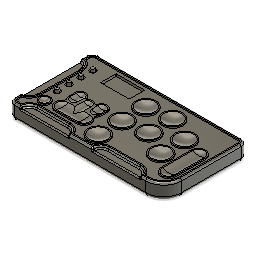
Pocket organ V11 mock-up v14 without engraving (Autodesk Fusion 360 design; units mm, degrees)
Autodesk Fusion 360 part; units mm, degrees
box "BoxPrimitive1" add length 70 width 130 height 13 placed x (0, 0, 1) y (1, 0, 0) z (0, 1, 0) at (0, 0, 0) makes body 1
fillet "Fillet1" radius 1.5 4 edges at (65, 13, 0) (130, 13, 35) (65, 13, 70) (0, 13, 35) on bodies 1
fillet "Fillet2" radius 3 4 edges at (65, 0, 70) (130, 0, 35) (65, 0, 0) (0, 0, 35) on bodies 1
fillet "Fillet3" radius 5 9 edges at (0.4393, 12.5607, 69.5607) (0, 7.25, 70) (0.8787, 0.8787, 69.1213) (0.4393, 12.5607, 0.4393) (0, 7.25, 0) (0.8787, 0.8787, 0.8787) (129.5607, 12.5607, 0.4393) (130, 7.25, 0) (129.1213, 0.8787, 0.8787) on bodies 1
fillet "Fillet4" radius 15 3 edges at (129.5607, 12.5607, 69.5607) (130, 7.25, 70) (129.1213, 0.8787, 69.1213) on bodies 1
sketch "keyboard top" plane through (0, 13, 0) normal (0, 1, 0) x (-1, 0, 0)
  arc A0 (-115, 68.5) -> (-128.5, 55) centre (-115, 55) ccw
  line L0 (-128.5, 55) -> (-128.5, 5)
  arc A1 (-128.5, 5) -> (-125, 1.5) centre (-125, 5) ccw
  line L1 (-125, 1.5) -> (-5, 1.5)
  arc A2 (-5, 1.5) -> (-1.5, 5) centre (-5, 5) ccw
  line L2 (-1.5, 5) -> (-1.5, 65)
  arc A3 (-1.5, 65) -> (-5, 68.5) centre (-5, 65) ccw
  line L3 (-5, 68.5) -> (-115, 68.5)
  line L4 (-25.5, 5) -> (-48.5, 5)
  line L5 (-49, 5.5) -> (-49, 17.5)
  line L6 (-48.5, 18) -> (-25.5, 18)
  line L7 (-25, 17.5) -> (-25, 5.5)
  line L8 (0.0001, 10) -> (0, 10)
  line L9 (-7, 17) -> (-7, 53)
  line L10 (0, 60) -> (0.0001, 60)
  arc A4 (-1.5, 59.8374) -> (-7, 53) centre (0, 53) ccw
  arc A5 (-1.5, 10.1626) -> (0, 10) centre (0, 17) ccw
  line L11 (0, 0) -> (-130, 0)
  line L12 (-130, 0) -> (-130, 70)
  line L13 (-130, 70) -> (0, 70)
  line L14 (0, 70) -> (0, 0)
  arc A6 (-49, 5.5) -> (-48.5, 5) centre (-48.5, 5.5) ccw
  arc A7 (-48.5, 18) -> (-49, 17.5) centre (-48.5, 17.5) ccw
  arc A8 (-25, 17.5) -> (-25.5, 18) centre (-25.5, 17.5) ccw
  arc A9 (-25.5, 5) -> (-25, 5.5) centre (-25.5, 5.5) ccw
  line L15 (-10, 69.9) -> (-10, 70)
  line L16 (-16.9, 63) -> (-43.1, 63)
  line L17 (-50, 69.9) -> (-50, 70)
  line L18 (-70, 69.9) -> (-70, 70)
  line L19 (-76.9, 63) -> (-103.1, 63)
  line L20 (-110, 69.9) -> (-110, 70)
  arc A10 (-110, 69.9) -> (-109.8565, 68.5) centre (-103.1, 69.9) ccw
  arc A11 (-76.9, 63) -> (-70.1435, 68.5) centre (-76.9, 69.9) ccw
  arc A12 (-50, 69.9) -> (-49.8565, 68.5) centre (-43.1, 69.9) ccw
  arc A13 (-10.1435, 68.5) -> (-10, 69.9) centre (-16.9, 69.9) ccw
  line L21 (-7, 0) -> (-13, 0)
  line L22 (-13, 0) -> (-13, 12.5)
  line L23 (-13, 12.5) -> (-13, 22.5)
  line L24 (-13, 22.5) -> (-13, 32.5)
  circle A14 centre (-13, 12.5) radius 2.5
  circle A15 centre (-13, 22.5) radius 2.5
  circle A16 centre (-13, 32.5) radius 2.5
  line L25 (-13, 32.5) -> (-13, 42.5)
  circle A17 centre (-13, 42.5) radius 2.5
  circle A18 centre (-13, 12.5) radius 1.5
  circle A19 centre (-13, 22.5) radius 1.5
  circle A20 centre (-13, 32.5) radius 1.5
  circle A21 centre (-13, 42.5) radius 1.5
  line L26 (-130, 0) -> (-102.5, 0)
  line L27 (-102.5, 0) -> (-82.5, 0)
  line L28 (-82.5, 0) -> (-62.5, 0)
  line L29 (-130, 0) -> (-119, 0)
  line L30 (-102.5, 0) -> (-102.5, 25)
  line L31 (-102.5, 25) -> (-102.5, 45)
  circle A22 centre (-102.5, 25) radius 7.5
  circle A23 centre (-102.5, 45) radius 7.5
  line L32 (-82.5, 0) -> (-82.5, 15)
  line L33 (-82.5, 15) -> (-82.5, 35)
  line L34 (-62.5, 0) -> (-62.5, 17.5)
  line L35 (-62.5, 17.5) -> (-62.5, 37.5)
  line L36 (-62.5, 37.5) -> (-62.5, 57.5)
  circle A24 centre (-82.5, 15) radius 7.5
  circle A25 centre (-82.5, 35) radius 7.5
  circle A26 centre (-62.5, 17.5) radius 7.5
  circle A27 centre (-62.5, 37.5) radius 7.5
  circle A28 centre (-62.5, 57.5) radius 7.5
  line L37 (-119, 30) -> (-119, 55) construction
  line L38 (0, 0) -> (-27, 0)
  line L39 (-27, 52) -> (-45, 52)
  line L40 (-27, 57) -> (-45, 57)
  arc A29 (-45, 57) -> (-45, 47) centre (-45, 52) ccw
  line L41 (-39.5, 47) -> (-32.5, 47)
  arc A30 (-27, 47) -> (-27, 57) centre (-27, 52) ccw
  line L42 (-27, 52) -> (-45, 52) construction
  line L43 (-36, 52) -> (-36, 40)
  line L44 (-45, 37) -> (-45, 42)
  line L45 (-27, 37) -> (-27, 42)
  line L46 (-32.5, 40) -> (-32.5, 47)
  arc A31 (-32.5, 52) -> (-39.5, 52) centre (-36, 52) ccw
  line L47 (-39.5, 52) -> (-39.5, 47)
  arc A32 (-39.5, 40) -> (-32.5, 40) centre (-36, 40) ccw
  line L48 (-36, 40) -> (-36, 52) construction
  line L49 (-41.5, 37) -> (-41.5, 42)
  arc A33 (-41.5, 42) -> (-48.5, 42) centre (-45, 42) ccw
  line L50 (-48.5, 42) -> (-48.5, 37)
  arc A34 (-48.5, 37) -> (-41.5, 37) centre (-45, 37) ccw
  line L51 (-45, 37) -> (-45, 42) construction
  line L52 (-23.5, 37) -> (-23.5, 42)
  arc A35 (-23.5, 42) -> (-30.5, 42) centre (-27, 42) ccw
  line L53 (-30.5, 42) -> (-30.5, 37)
  arc A36 (-30.5, 37) -> (-23.5, 37) centre (-27, 37) ccw
  line L54 (-27, 37) -> (-27, 42) construction
  line L55 (-114, 30) -> (-114, 55)
  arc A37 (-114, 55) -> (-124, 55) centre (-119, 55) ccw
  line L56 (-124, 55) -> (-124, 30)
  arc A38 (-124, 30) -> (-114, 30) centre (-119, 30) ccw
  line L57 (-119, 30) -> (-119, 55) construction
  line L58 (-27, 52) -> (-15, 52)
  line L59 (-15, 52) -> (-15, 55)
  circle A39 centre (-15, 55) radius 3.5
  line L60 (-119, 55) -> (-119, 30)
  line L61 (-45, 37) -> (-45, 42)
  line L62 (-27, 37) -> (-27, 42)
  line L63 (-49.8565, 68.5) -> (-70.1435, 68.5)
  line L64 (-109.8565, 68.5) -> (-115, 68.5)
  line L65 (-128.5, 55) -> (-128.5, 5)
  line L66 (-125, 1.5) -> (-5, 1.5)
  line L67 (-1.5, 10.1626) -> (-1.5, 5)
  line L68 (-1.5, 59.8374) -> (-1.5, 65)
  line L69 (-10.1435, 68.5) -> (-5, 68.5)
  arc A40 (-1.5, 65) -> (-5, 68.5) centre (-5, 65) ccw
  arc A41 (-5, 1.5) -> (-1.5, 5) centre (-5, 5) ccw
  arc A42 (-128.5, 5) -> (-125, 1.5) centre (-125, 5) ccw
  arc A43 (-115, 68.5) -> (-128.5, 55) centre (-115, 55) ccw
  arc A44 (-109.8565, 68.5) -> (-103.1, 63) centre (-103.1, 69.9) ccw
  arc A45 (-70.1435, 68.5) -> (-70, 69.9) centre (-76.9, 69.9) ccw
  arc A46 (-49.8565, 68.5) -> (-43.1, 63) centre (-43.1, 69.9) ccw
  arc A47 (-16.9, 63) -> (-10.1435, 68.5) centre (-16.9, 69.9) ccw
  arc A48 (0, 60) -> (-1.5, 59.8374) centre (0, 53) ccw
  arc A49 (-7, 17) -> (-1.5, 10.1626) centre (0, 17) ccw
  arc A50 (-110.6266, 67.5) -> (-103.1, 62) centre (-103.1, 69.9) ccw
  line L70 (-76.9, 62) -> (-103.1, 62)
  arc A51 (-76.9, 62) -> (-69.3734, 67.5) centre (-76.9, 69.9) ccw
  line L71 (-50.6266, 67.5) -> (-69.3734, 67.5)
  arc A52 (-50.6266, 67.5) -> (-43.1, 62) centre (-43.1, 69.9) ccw
  line L72 (-16.9, 62) -> (-43.1, 62)
  arc A53 (-16.9, 62) -> (-9.3734, 67.5) centre (-16.9, 69.9) ccw
  line L73 (-9.3734, 67.5) -> (-5, 67.5)
  arc A54 (-2.5, 65) -> (-5, 67.5) centre (-5, 65) ccw
  line L74 (-2.5, 60.5993) -> (-2.5, 65)
  arc A55 (-2.5, 60.5993) -> (-8, 53) centre (0, 53) ccw
  line L75 (-8, 17) -> (-8, 53)
  arc A56 (-8, 17) -> (-2.5, 9.4007) centre (0, 17) ccw
  line L76 (-2.5, 9.4007) -> (-2.5, 5)
  arc A57 (-5, 2.5) -> (-2.5, 5) centre (-5, 5) ccw
  line L77 (-125, 2.5) -> (-5, 2.5)
  arc A58 (-127.5, 5) -> (-125, 2.5) centre (-125, 5) ccw
  line L78 (-127.5, 55) -> (-127.5, 5)
  arc A59 (-115, 67.5) -> (-127.5, 55) centre (-115, 55) ccw
  line L79 (-110.6266, 67.5) -> (-115, 67.5)
  line L80 (-125, 55) -> (-125, 30)
  arc A60 (-125, 30) -> (-113, 30) centre (-119, 30) ccw
  line L81 (-113, 30) -> (-113, 55)
  arc A61 (-113, 55) -> (-125, 55) centre (-119, 55) ccw
  circle A62 centre (-102.5, 25) radius 8.5
  circle A63 centre (-102.5, 45) radius 8.5
  circle A64 centre (-82.5, 35) radius 8.5
  circle A65 centre (-82.5, 15) radius 8.5
  circle A66 centre (-62.5, 17.5) radius 8.5
  circle A67 centre (-62.5, 37.5) radius 8.5
  circle A68 centre (-62.5, 57.5) radius 8.5
  line L82 (-40.5, 40) -> (-40.5, 42)
  arc A69 (-40.5, 42) -> (-46.5827, 46.2125) centre (-45, 42) ccw
  line L83 (-49.5, 42) -> (-49.5, 37)
  arc A70 (-49.5, 37) -> (-40.5, 37) centre (-45, 37) ccw
  arc A71 (-25.4173, 46.2125) -> (-31.5, 42) centre (-27, 42) ccw
  line L84 (-31.5, 42) -> (-31.5, 40)
  arc A72 (-31.5, 37) -> (-22.5, 37) centre (-27, 37) ccw
  line L85 (-22.5, 37) -> (-22.5, 42)
  circle A73 centre (-15, 55) radius 4.5
  line L86 (-39.5, 47) -> (-39.5, 40)
  line L87 (-32.5, 47) -> (-32.5, 52)
  line L88 (-32.5, 47) -> (-27, 47)
  line L89 (-45, 47) -> (-39.5, 47)
  line L90 (-40.5, 46) -> (-40.5, 40)
  line L91 (-31.5, 40) -> (-31.5, 46)
  line L92 (-31.5, 46) -> (-27, 46)
  line L93 (-27, 58) -> (-45, 58)
  arc A74 (-46.5827, 46.2125) -> (-45, 46) centre (-45, 52) ccw
  line L94 (-45, 46) -> (-40.5, 46)
  arc A75 (-45, 58) -> (-48.893, 47.4344) centre (-45, 52) ccw
  arc A76 (-48.5935, 44.7087) -> (-49.5, 42) centre (-45, 42) ccw
  line L95 (-40.5, 37) -> (-40.5, 40)
  line L96 (-31.5, 40) -> (-31.5, 37)
  arc A77 (-27, 46) -> (-25.4173, 46.2125) centre (-27, 52) ccw
  arc A78 (-21, 52) -> (-27, 58) centre (-27, 52) ccw
  arc A79 (-23.107, 47.4344) -> (-21, 52) centre (-27, 52) ccw
  arc A80 (-22.5, 42) -> (-23.4065, 44.7087) centre (-27, 42) ccw
  arc A81 (-23.107, 47.4344) -> (-23.4065, 44.7087) centre (-21.8094, 45.9125) ccw
  arc A82 (-48.5935, 44.7087) -> (-48.893, 47.4344) centre (-50.1906, 45.9125) ccw
  line L97 (-31.5, 37) -> (-32.6459, 37)
  line L98 (-40.5, 37) -> (-39.3541, 37)
  arc A83 (-40.5, 40) -> (-39.3541, 37) centre (-36, 40) ccw
  arc A84 (-32.6459, 37) -> (-31.5, 40) centre (-36, 40) ccw
  arc A85 (-39.3541, 37) -> (-32.6459, 37) centre (-36, 40) ccw
  arc A86 (-111.6703, 67.5) -> (-103.1, 61) centre (-103.1, 69.9) ccw
  line L99 (-76.9, 61) -> (-103.1, 61)
  arc A87 (-76.9, 61) -> (-68.3297, 67.5) centre (-76.9, 69.9) ccw
  arc A88 (-51.6703, 67.5) -> (-43.1, 61) centre (-43.1, 69.9) ccw
  line L100 (-16.9, 61) -> (-43.1, 61)
  arc A89 (-16.9, 61) -> (-8.3297, 67.5) centre (-16.9, 69.9) ccw
  arc A90 (-2.5, 61.6458) -> (-9, 53) centre (0, 53) ccw
  line L101 (-9, 17) -> (-9, 53)
  arc A91 (-9, 17) -> (-2.5, 8.3542) centre (0, 17) ccw
  line L102 (-28.4325, 53.5487) -> (-44.8065, 53.5487) construction
  line L103 (-44.8065, 53.5487) -> (-44.8065, 47.5487) construction
  line L104 (-44.8065, 47.5487) -> (-28.4325, 47.5487) construction
  line L105 (-28.4325, 47.5487) -> (-28.4325, 53.5487) construction
  line L106 (-59.4724, 21.1298) -> (-65.7077, 21.1298) construction
  line L107 (-65.7077, 21.1298) -> (-65.7077, 11.1298) construction
  line L108 (-65.7077, 11.1298) -> (-59.4724, 11.1298) construction
  line L109 (-59.4724, 11.1298) -> (-59.4724, 21.1298) construction
  line L110 (-79.7168, 18.5949) -> (-85.7178, 18.5949) construction
  line L111 (-85.7178, 18.5949) -> (-85.7178, 8.5949) construction
  line L112 (-85.7178, 8.5949) -> (-79.7168, 8.5949) construction
  line L113 (-79.7168, 8.5949) -> (-79.7168, 18.5949) construction
  line L114 (-99.8243, 28.6873) -> (-105.2686, 28.6873) construction
  line L115 (-105.2686, 28.6873) -> (-105.2686, 18.6873) construction
  line L116 (-105.2686, 18.6873) -> (-99.8243, 18.6873) construction
  line L117 (-99.8243, 18.6873) -> (-99.8243, 28.6873) construction
  line L118 (-60.2821, 41.2383) -> (-65.1893, 41.2383) construction
  line L119 (-65.1893, 41.2383) -> (-65.1893, 31.2383) construction
  line L120 (-65.1893, 31.2383) -> (-60.2821, 31.2383) construction
  line L121 (-60.2821, 31.2383) -> (-60.2821, 41.2383) construction
  line L122 (-79.041, 38.5391) -> (-85.7354, 38.5391) construction
  line L123 (-85.7354, 38.5391) -> (-85.7354, 28.5391) construction
  line L124 (-85.7354, 28.5391) -> (-79.041, 28.5391) construction
  line L125 (-79.041, 28.5391) -> (-79.041, 38.5391) construction
  line L126 (-98.874, 48.4203) -> (-106.0566, 48.4203) construction
  line L127 (-106.0566, 48.4203) -> (-106.0566, 38.4203) construction
  line L128 (-106.0566, 38.4203) -> (-98.874, 38.4203) construction
  line L129 (-98.874, 38.4203) -> (-98.874, 48.4203) construction
  line L130 (-59.6073, 61.3467) -> (-65.6034, 61.3467) construction
  line L131 (-65.6034, 61.3467) -> (-65.6034, 51.3467) construction
  line L132 (-65.6034, 51.3467) -> (-59.6073, 51.3467) construction
  line L133 (-59.6073, 51.3467) -> (-59.6073, 61.3467) construction
  line L134 (-116.6195, 46.4025) -> (-121.9759, 46.4025) construction
  line L135 (-121.9759, 46.4025) -> (-121.9759, 36.4025) construction
  line L136 (-121.9759, 36.4025) -> (-116.6195, 36.4025) construction
  line L137 (-116.6195, 36.4025) -> (-116.6195, 46.4025) construction
  line L138 (-14.0627, 56.7468) -> (-16.382, 56.7468) construction
  line L139 (-16.382, 56.7468) -> (-16.382, 51.7468) construction
  line L140 (-16.382, 51.7468) -> (-14.0627, 51.7468) construction
  line L141 (-14.0627, 51.7468) -> (-14.0627, 56.7468) construction
  line L142 (-25.6408, 36.5912) -> (-25.6408, 42.4115) construction
  line L143 (-25.6408, 42.4115) -> (-29.6408, 42.4115) construction
  line L144 (-29.6408, 42.4115) -> (-29.6408, 36.5912) construction
  line L145 (-29.6408, 36.5912) -> (-25.6408, 36.5912) construction
  line L146 (-34.3337, 38.9989) -> (-34.3337, 44.5516) construction
  line L147 (-34.3337, 44.5516) -> (-38.3337, 44.5516) construction
  line L148 (-38.3337, 44.5516) -> (-38.3337, 38.9989) construction
  line L149 (-38.3337, 38.9989) -> (-34.3337, 38.9989) construction
  line L150 (-43.8694, 36.5932) -> (-43.8694, 42.1537) construction
  line L151 (-43.8694, 42.1537) -> (-47.8694, 42.1537) construction
  line L152 (-47.8694, 42.1537) -> (-47.8694, 36.5932) construction
  line L153 (-47.8694, 36.5932) -> (-43.8694, 36.5932) construction
  point P0 (-25, 5)
  point P1 (-49, 5)
  point P2 (-25, 18)
  point P3 (-10, 63)
  point P4 (-50, 63)
  point P5 (-70, 63)
  point P6 (-110, 63)
  dimension "d10" = 24
  dimension "d11" = 13
  dimension "d12" = 7
  dimension "d13" = 7
  dimension "d18" = 0.5
  dimension "d21" = 40
  dimension "d22" = 40
  dimension "d23" = 6.9
  dimension "d28" = 6
  dimension "d29" = 12.5
  dimension "d30" = 10
  dimension "d31" = 10
  dimension "d32" = 5
  dimension "d33" = 5
  dimension "d34" = 5
  dimension "d35" = 10
  dimension "d36" = 5
  dimension "d37" = 3
  dimension "d38" = 3
  dimension "d39" = 3
  dimension "d40" = 3
  dimension "d46" = 27.5
  dimension "d47" = 20
  dimension "d48" = 20
  dimension "d49" = 11
  dimension "d50" = 55
  dimension "d51" = 25
  dimension "d52" = 20
  dimension "d53" = 15
  dimension "d54" = 15
  dimension "d55" = 15
  dimension "d56" = 20
  dimension "d57" = 17.5
  dimension "d58" = 20
  dimension "d59" = 20
  dimension "d60" = 15
  dimension "d61" = 15
  dimension "d62" = 15
  dimension "d63" = 15
  dimension "d64" = 15
  dimension "d65" = 30
  dimension "d74" = 27
  dimension "d75" = 52
  dimension "d76" = 18
  dimension "d77" = 10
  dimension "d78" = 15
  dimension "d79" = 5
  dimension "d80" = 15
  dimension "d81" = 5
  dimension "d82" = 7
  dimension "d83" = 7
  dimension "d84" = 7
  dimension "d86" = 10
  dimension "d87" = 7
  dimension "d120" = 1
  dimension "d121" = 1
  dimension "d122" = 1
  dimension "d123" = 1
  dimension "d124" = 1
  dimension "d125" = 1
  dimension "d126" = 1
  dimension "d127" = 1
  dimension "d128" = 1
  dimension "d131" = 1
  dimension "d133" = 2
  dimension "d134" = 2
  constraint horizontal L4
  constraint vertical L5
  constraint horizontal L6
  constraint vertical L7
  constraint tangent L9 A4
  constraint tangent L10 A4
  constraint tangent L8 A5
  constraint tangent L9 A5
  constraint horizontal L11
  constraint vertical L12
  constraint horizontal L13
  constraint vertical L14
  constraint coincident L11.start L14.end
  constraint coincident P1 L4
  constraint coincident P1 L5
  constraint tangent L4 A6
  constraint tangent L5 A6
  constraint tangent L5 A7
  constraint tangent L6 A7
  constraint equal A6 A7
  constraint coincident P2 L6
  constraint coincident P2 L7
  constraint tangent L6 A8
  constraint tangent L7 A8
  constraint equal A6 A8
  constraint coincident P0 L4
  constraint coincident P0 L7
  constraint tangent L4 A9
  constraint tangent L7 A9
  constraint equal A6 A9
  constraint coincident L13 L15.end
  constraint perpendicular L13 L15
  constraint perpendicular L15 L16
  constraint coincident L13 L17.end
  constraint perpendicular L13 L17
  constraint coincident L13 L18.end
  constraint perpendicular L13 L18
  constraint horizontal L19
  constraint coincident L13 L20.end
  constraint perpendicular L13 L20
  constraint coincident P6 L19
  constraint coincident P6 L20
  constraint tangent L19 A10
  constraint tangent L20 A10
  constraint coincident P5 L18
  constraint coincident P5 L19
  constraint tangent L18 A11
  constraint tangent L19 A11
  constraint equal A10 A11
  constraint coincident P4 L16
  constraint coincident P4 L17
  constraint tangent L16 A12
  constraint tangent L17 A12
  constraint equal A10 A12
  constraint coincident P3 L15
  constraint coincident P3 L16
  constraint tangent L15 A13
  constraint tangent L16 A13
  constraint equal A10 A13
  constraint coincident L11 L21.start
  constraint coincident L11 L21.end
  constraint perpendicular L21 L22
  constraint perpendicular L1 L23
  constraint coincident L22.end L23.start
  constraint coincident L23.end L24.start
  constraint coincident L24.end A16.centre
  constraint coincident L25.end A17.centre
  constraint concentric A14 A18
  constraint concentric A15 A19
  constraint concentric A16 A20
  constraint concentric A17 A21
  constraint perpendicular L12 L26
  constraint parallel L11 L27
  constraint parallel L11 L28
  constraint perpendicular L12 L29
  constraint perpendicular L1 L30
  constraint coincident L30.end L31.start
  constraint coincident L31.end A23.centre
  constraint perpendicular L1 L32
  constraint perpendicular L11 L34
  constraint coincident L32.end L33.start
  constraint coincident L33.end A25.centre
  constraint coincident L34.end L35.start
  constraint coincident L35.end L36.start
  constraint coincident L36.end A28.centre
  constraint perpendicular L14 L38
  constraint tangent L40 A29
  constraint tangent A29 L41
  constraint parallel L40 L41
  constraint tangent L41 A30
  constraint tangent L40 A30
  constraint coincident L39.end A29.centre
  constraint coincident L39.start A30.centre
  constraint midpoint L39 L43.start
  constraint perpendicular L39 L43
  constraint tangent L46 A31
  constraint tangent A31 L47
  constraint parallel L46 L47
  constraint tangent L47 A32
  constraint tangent L46 A32
  constraint coincident L43.start A31.centre
  constraint perpendicular L39 L48
  constraint coincident L43.end A32.centre
  constraint tangent L49 A33
  constraint tangent A33 L50
  constraint parallel L49 L50
  constraint tangent L50 A34
  constraint tangent L49 A34
  constraint coincident L44.end A33.centre
  constraint coincident L44.start A34.centre
  constraint tangent L52 A35
  constraint tangent A35 L53
  constraint parallel L52 L53
  constraint tangent L53 A36
  constraint tangent L52 A36
  constraint coincident L45.end A35.centre
  constraint coincident L45.start A36.centre
  constraint tangent L55 A37
  constraint tangent A37 L56
  constraint parallel L55 L56
  constraint tangent L56 A38
  constraint tangent L55 A38
  constraint coincident L37.end A37.centre
  constraint coincident L37.start A38.centre
  constraint perpendicular L58 L59
  constraint coincident L59.end A39.centre
  constraint coincident L3 A12.end
  constraint coincident L3 A11.end
  constraint coincident L3 A10.end
  constraint coincident A0.start L3.end
  constraint coincident A0.end L0.start
  constraint coincident L0.end A1.start
  constraint coincident A1.end L1.start
  constraint coincident L1.end A2.start
  constraint coincident L2 A5.start
  constraint coincident A2.end L2.start
  constraint coincident L2 A4.start
  constraint coincident L2.end A3.start
  constraint coincident L3 A13.start
  constraint coincident A3.end L3.start
  constraint tangent L0 A42
  constraint tangent L64 A43
  constraint concentric A10 A44
  constraint concentric A11 A45
  constraint concentric A12 A46
  constraint concentric A13 A47
  constraint concentric A4 A48
  constraint concentric A5 A49
  constraint tangent A31 L86
  constraint parallel L46 L86
  constraint parallel L47 L87
  constraint tangent A29 L88
  constraint parallel L40 L89
  constraint parallel L86 L90
  constraint concentric A32 A83
  constraint parallel L46 L91
  constraint parallel L88 L92
  constraint concentric A30 A77
  constraint parallel L40 L93
  constraint concentric A29 A74
  constraint parallel L89 L94
  constraint tangent L91 A83
  constraint tangent L90 A83
  constraint tangent A74 L94
  constraint tangent L92 A77
  constraint tangent L93 A77
  constraint tangent L93 A74
  constraint concentric A74 A75
  constraint parallel L49 L82
  constraint concentric A33 A69
  constraint parallel L50 L83
  constraint concentric A34 A70
  constraint tangent L82 A70
  constraint tangent L82 A69
  constraint tangent A69 L83
  constraint tangent L83 A70
  constraint concentric A69 A76
  constraint parallel L49 L95
  constraint tangent A69 L95
  constraint concentric A35 A71
  constraint parallel L53 L84
  constraint concentric A36 A72
  constraint parallel L52 L85
  constraint tangent A71 L85
  constraint tangent L84 A72
  constraint tangent A71 L84
  constraint tangent A72 L85
  constraint parallel L53 L96
  constraint tangent A71 L96
  constraint coincident L58 A78.start
  constraint concentric A77 A78
  constraint concentric A77 A79
  constraint concentric A71 A80
  constraint tangent A80 A81
  constraint tangent A79 A81
  constraint tangent A76 A82
  constraint tangent A75 A82
  constraint coincident L97.end A83
  constraint perpendicular L96 L97
  constraint perpendicular L95 L98
  constraint concentric A83 A84
  constraint concentric A83 A85
  constraint concentric A4 A90
  constraint parallel L9 L101
  constraint concentric A49 A91
  constraint tangent L101 A91
  constraint tangent A90 L101
  constraint coincident L76 A91.end
  constraint coincident L74 A90.start
  constraint concentric A46 A88
  constraint parallel L16 L100
  constraint concentric A47 A89
  constraint tangent A88 L100
  constraint tangent L100 A89
  constraint coincident L73 A89.end
  constraint coincident L71 A88.start
  constraint concentric A44 A86
  constraint parallel L19 L99
  constraint concentric A11 A87
  constraint tangent A86 L99
  constraint tangent L99 A87
  constraint coincident L71 A87.end
  constraint coincident L79 A86.start
  constraint perpendicular L102 L103
  constraint parallel L102 L104
  constraint parallel L103 L105
  constraint perpendicular L106 L107
  constraint parallel L106 L108
  constraint parallel L107 L109
  constraint perpendicular L110 L111
  constraint parallel L110 L112
  constraint parallel L111 L113
  constraint perpendicular L114 L115
  constraint parallel L114 L116
  constraint parallel L115 L117
  constraint perpendicular L118 L119
  constraint parallel L118 L120
  constraint parallel L119 L121
  constraint perpendicular L122 L123
  constraint parallel L122 L124
  constraint parallel L123 L125
  constraint perpendicular L126 L127
  constraint parallel L126 L128
  constraint parallel L127 L129
  constraint perpendicular L130 L131
  constraint parallel L130 L132
  constraint parallel L131 L133
  constraint perpendicular L134 L135
  constraint parallel L134 L136
  constraint parallel L135 L137
  constraint perpendicular L138 L139
  constraint parallel L138 L140
  constraint parallel L139 L141
  constraint perpendicular L142 L143
  constraint parallel L142 L144
  constraint parallel L143 L145
  constraint perpendicular L146 L147
  constraint parallel L146 L148
  constraint parallel L147 L149
  constraint perpendicular L150 L151
  constraint parallel L150 L152
  constraint parallel L151 L153
  measures "d10" distance of P0 P1
  measures "d11" distance of P0 P2
  measures "d12" radius of A4
  measures "d13" radius of A5
  measures "d18" radius of A6
  measures "d21" distance of P3 P4
  measures "d22" distance of P5 P6
  measures "d23" radius of A10
  measures "d28" distance of L21.start L21.end
  measures "d29" distance of L21.end L22.end
  measures "d30" distance of L22.end L23.end
  measures "d31" distance of L23.end L24.end
  measures "d32" diameter of A14
  measures "d33" diameter of A15
  measures "d34" diameter of A16
  measures "d35" distance of L24.end L25.end
  measures "d36" diameter of A17
  measures "d37" diameter of A18
  measures "d38" diameter of A19
  measures "d39" diameter of A20
  measures "d40" diameter of A21
  measures "d46" distance of L11.end L26.end
  measures "d47" distance of L26.end L27.end
  measures "d48" distance of L27.end L28.end
  measures "d49" distance of L11.end L29.end
  measures "d50" distance of L29.end L37.end
  measures "d51" distance of L26.end L30.end
  measures "d52" distance of L30.end L31.end
  measures "d53" diameter of A22
  measures "d54" diameter of A23
  measures "d55" distance of L27.end L32.end
  measures "d56" distance of L32.end L33.end
  measures "d57" distance of L28.end L34.end
  measures "d58" distance of L34.end L35.end
  measures "d59" distance of L35.end L36.end
  measures "d60" diameter of A24
  measures "d61" diameter of A25
  measures "d62" diameter of A26
  measures "d63" diameter of A27
  measures "d64" diameter of A28
  measures "d65" distance of L29.end L37.start
  measures "d74" distance of L11.start L38.end
  measures "d75" distance of L38.end L39.start
  measures "d76" distance of L39.start L39.end
  measures "d77" diameter of A29
  measures "d78" distance of L39.end L44.start
  measures "d79" distance of L44.start L44.end
  measures "d80" distance of L39.start L45.start
  measures "d81" distance of L45.start L45.end
  measures "d82" diameter of A31
  measures "d83" diameter of A33
  measures "d84" diameter of A35
  measures "d86" diameter of A37
  measures "d87" diameter of A39
  measures "d133" radius of A81
  measures "d134" radius of A82
extrude "Extrude1" cut sketch "keyboard top" against normal blind 2 contours L2 A5 L14 A48 | L2 L9 A4 A49 bodies 1
fillet "Fillet5" radius 1 8 edges at (0, 11.25, 10) (0.4432, 12.5645, 10.014) (5.4544, 13, 12.6125) (7, 13, 35) (5.4544, 13, 57.3875) (0.4432, 12.5645, 59.986) (0, 11.25, 60) (0, 11, 35) on bodies 1
fillet "Fillet6" radius 1 7 edges at (0.25, 10.6614, 9.7242) (0.938, 10.998, 10.0631) (5.2915, 11, 12.4174) (7, 11, 35) (5.2915, 11, 57.5826) (0.938, 10.998, 59.9369) (0.25, 10.6614, 60.2758) on bodies 1
extrude "Extrude2" cut sketch "keyboard top" against normal blind 3 contours L4 L5 L6 L7 A6 A7 A8 A9 bodies 1
extrude "Extrude3" cut sketch "keyboard top" against normal blind 2 contours L3 L13 L18 L20 A10 A45 | L3 L19 A11 A44 | L3 L13 L15 L17 A12 A13 | L3 L16 A46 A47 bodies 1
fillet "Fillet7" radius 1 20 edges at (10, 11.25, 70) (10, 11.7739, 69.9748) (10.0221, 12.7363, 69.3487) (12.544, 13, 64.5488) (30, 13, 63) (47.456, 13, 64.5488) (49.9779, 12.7363, 69.3487) (50, 11.7739, 69.9748) (50, 11.25, 70) (30, 11, 70) (70, 11.25, 70) (70, 11.7739, 69.9748) (70.0221, 12.7363, 69.3487) (72.544, 13, 64.5488) (90, 13, 63) (107.456, 13, 64.5488) (109.9779, 12.7363, 69.3487) (110, 11.7739, 69.9748) (110, 11.25, 70) (90, 11, 70) on bodies 1
fillet "Fillet8" radius 1 14 edges at (9.717, 10.6656, 69.7463) (10.0518, 10.9984, 69.0566) (12.3503, 11, 64.7125) (30, 11, 63) (47.6497, 11, 64.7125) (49.9482, 10.9984, 69.0566) (50.283, 10.6656, 69.7463) (69.717, 10.6656, 69.7463) (70.0518, 10.9984, 69.0566) (72.3503, 11, 64.7125) (90, 11, 63) (107.6497, 11, 64.7125) (109.9482, 10.9984, 69.0566) (110.283, 10.6656, 69.7463) on bodies 1
extrude "Extrude4" cut sketch "keyboard top" against normal blind 1.5 contours L22 L23 A14 A18 | L22 L23 A14 A18 | L23 L24 A15 A19 | L23 L24 A15 A19 | L24 A16 L25 A20 | L24 A16 L25 A20 | A17 bodies 1
extrude "Extrude5" add sketch "keyboard top" along normal blind 2 contours L22 L23 A18 | L22 L23 A18 | L23 L24 A19 | L23 L24 A19 | L24 L25 A20 | L24 L25 A20 | A21 bodies 1
fillet "Fillet9" radius 1 4 edges at (14.3985, 15, 11.9576) (14.3985, 15, 21.9576) (14.3985, 15, 31.9576) (14.3985, 15, 41.9576) on bodies 1
sphere "SpherePrimitive1" add diameter 39 placed x (-1, 0, 0) y (0, 0, 1) z (0, 1, 0) at (62.5, 13, 17.5) separate body makes body 2
sphere "SpherePrimitive2" add diameter 39 placed x (-1, 0, 0) y (0, 0, 1) z (0, 1, 0) at (62.5, 13, 37.5) bodies 2
sphere "SpherePrimitive3" add diameter 39 placed x (-1, 0, 0) y (0, 0, 1) z (0, 1, 0) at (62.5, 13, 57.5) bodies 2
sphere "SpherePrimitive4" add diameter 39 placed x (-1, 0, 0) y (0, 0, 1) z (0, 1, 0) at (82.5, 13, 15) bodies 2
sphere "SpherePrimitive5" add diameter 39 placed x (-1, 0, 0) y (0, 0, 1) z (0, 1, 0) at (82.5, 13, 35) bodies 2
sphere "SpherePrimitive6" add diameter 39 placed x (-1, 0, 0) y (0, 0, 1) z (0, 1, 0) at (102.5, 13, 25) bodies 2
sphere "SpherePrimitive7" add diameter 39 placed x (-1, 0, 0) y (0, 0, 1) z (0, 1, 0) at (102.5, 13, 45) bodies 2
move_body "Move1" bodies 2 to x (1, 0, 0) y (0, 1, 0) z (0, 0, 1) at (0, 18, 0)
combine "Combine1" operation cut target body 1 tool bodies 2 keep tools
sphere "SpherePrimitive9" add diameter 26 placed x (-1, 0, 0) y (0, 0, 1) z (0, 1, 0) at (119, 13, 55) separate body makes body 3
sphere "SpherePrimitive10" add diameter 26 placed x (-1, 0, 0) y (0, 0, 1) z (0, 1, 0) at (119, 13, 30) separate body makes body 4
pipe "Pipe1" add diameter 26 path "keyboard top" along L60 bodies 3 4 merging no bodies
combine "Combine2" operation add target body 3 tool bodies 4 keep tools
combine "Combine3" operation add target body 3 tool bodies 4
move_body "Move2" bodies 3 to x (1, 0, 0) y (0, 1, 0) z (0, 0, 1) at (0, 12, 0)
combine "Combine4" operation cut target body 1 tool bodies 3 keep tools
sphere "SpherePrimitive11" add diameter 26 placed x (-1, 0, 0) y (0, 0, 1) z (0, 1, 0) at (27, 13, 52) separate body makes body 5
sphere "SpherePrimitive12" add diameter 26 placed x (-1, 0, 0) y (0, 0, 1) z (0, 1, 0) at (45, 13, 52) separate body makes body 6
pipe "Pipe2" add diameter 26 path "keyboard top" along L39 bodies 5 6 merging no bodies
combine "Combine5" operation add target body 5 tool bodies 6
move_body "Move3" bodies 5 to x (1, 0, 0) y (0, 1, 0) z (0, 0, 1) at (0, 12, 0)
sphere "SpherePrimitive13" add diameter 13.25 placed x (-1, 0, 0) y (0, 0, 1) z (0, 1, 0) at (27, 13, 42) separate body makes body 7
sphere "SpherePrimitive14" add diameter 13.25 placed x (-1, 0, 0) y (0, 0, 1) z (0, 1, 0) at (36, 13, 52) separate body makes body 8
sphere "SpherePrimitive15" add diameter 13.25 placed x (-1, 0, 0) y (0, 0, 1) z (0, 1, 0) at (45, 13, 42) separate body makes body 9
sphere "SpherePrimitive16" add diameter 13.25 placed x (-1, 0, 0) y (0, 0, 1) z (0, 1, 0) at (36, 13, 40) bodies 7 8 9
sphere "SpherePrimitive17" add diameter 13.25 placed x (-1, 0, 0) y (0, 0, 1) z (0, 1, 0) at (27, 13, 37) bodies 7
sphere "SpherePrimitive18" add diameter 13.25 placed x (-1, 0, 0) y (0, 0, 1) z (0, 1, 0) at (45, 13, 37) bodies 7
pipe "Pipe3" add diameter 13.25 path "keyboard top" along L43 bodies 7
pipe "Pipe4" add diameter 13.25 path "keyboard top" along L61 bodies 7
pipe "Pipe5" add diameter 13.25 path "keyboard top" along L45 bodies 7
move_body "Move4" bodies 7 to x (1, 0, 0) y (0, 1, 0) z (0, 0, 1) at (0, 5.625, 0)
sphere "SpherePrimitive19" add diameter 13.25 placed x (-1, 0, 0) y (0, 0, 1) z (0, 1, 0) at (15, 13, 55) separate body makes body 10
move_body "Move5" bodies 10 to x (1, 0, 0) y (0, 1, 0) z (0, 0, 1) at (0, 5.625, 0)
combine "Combine6" operation cut target body 1 tool bodies 7 5 10 keep tools
extrude "Extrude6" cut sketch "keyboard top" against normal blind 1 contours L71 L73 A54 L74 L76 A57 L77 A58 L78 A59 L79 A86 L99 A87 A88 L100 A89 A90 L101 A91 bodies 1
sketch "Sketch22" plane through (0, 11, 0) normal (0, 1, 0) x (-1, 0, 0)
  spline S0 degree 3 poles (-1.125, 58.8936) (-1.0834, 58.9015) (-1.0417, 58.909) (-1, 58.9163) knots 0 0 0 0 0.012705 0.012705 0.012705 0.012705
  arc A0 (-1.125, 58.8936) -> (-6, 53) centre (0, 53) ccw
  line L0 (-6, 53) -> (-6, 17)
  arc A1 (-6, 17) -> (-1.125, 11.1064) centre (0, 17) ccw
  spline S1 degree 3 poles (-1, 11.0837) (-1.0417, 11.091) (-1.0834, 11.0985) (-1.125, 11.1064) knots 0.308282 0.308282 0.308282 0.308282 0.320987 0.320987 0.320987 0.320987
  line L1 (-1, 11.0837) -> (-1, 58.9163)
  line L2 (-1.8664, 27.0776) -> (-1.8664, 41.0816) construction
  line L3 (-1.8664, 41.0816) -> (-5.8664, 41.0816) construction
  line L4 (-5.8664, 41.0816) -> (-5.8664, 27.0776) construction
  line L5 (-5.8664, 27.0776) -> (-1.8664, 27.0776) construction
  line L6 (-17.7057, 68.7788) -> (-41.6647, 68.7788) construction
  line L7 (-41.6647, 68.7788) -> (-41.6647, 64.7788) construction
  line L8 (-41.6647, 64.7788) -> (-17.7057, 64.7788) construction
  line L9 (-17.7057, 64.7788) -> (-17.7057, 68.7788) construction
  line L10 (-78.1661, 68.6438) -> (-102.5743, 68.6438) construction
  line L11 (-102.5743, 68.6438) -> (-102.5743, 64.6438) construction
  line L12 (-102.5743, 64.6438) -> (-78.1661, 64.6438) construction
  line L13 (-78.1661, 64.6438) -> (-78.1661, 68.6438) construction
  constraint perpendicular L2 L3
  constraint parallel L2 L4
  constraint parallel L3 L5
  constraint perpendicular L6 L7
  constraint parallel L6 L8
  constraint parallel L7 L9
  constraint perpendicular L10 L11
  constraint parallel L10 L12
  constraint parallel L11 L13
extrude "Extrude7" [rolled back] along distance -1 taper angle 0
extrude "Extrude8" [rolled back] along distance -1 taper angle 0
extrude "Extrude9" [rolled back] along distance -1.5 taper angle 0
extrude "Extrude10" [rolled back] along distance -1 taper angle 0
hidden bodies 2 3 5 7 10
named bodies: "enclosure", "AB key depression", "Sharp key depression", "Minor key depression", "alterations key depression", "Melody key depression"
